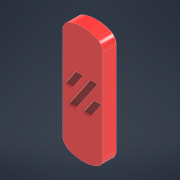
# Autodesk Inventor part: Cover_Square
Saved by Autodesk Inventor 2022.1 (Build 261234000, 234)
## iProperties
Created: 2021-09-01
Part Number: Cover_Square
Material: Generisch
Document SubType Name: Modeling
Designer: Rama
Density: 1 g/cm^3
Appearance: Hellrot
Author: Rama
Autodesk Inventor part; units mm, degrees
ref_plane "YZ Plane" through (0, 0, 0) normal (1, 0, 0) x (0, 1, 0)
ref_plane "XZ Plane" through (0, 0, 0) normal (0, 1, 0) x (-1, 0, 0)
sketch "Skizze1" plane through (0, 0, 0) normal (0, 0, 1) x (1, 0, 0)
  line L0 (7.75, -17.6806) -> (7.75, 17.6806) projected
  line L1 (-7.75, 17.6806) -> (-7.75, -17.6806) projected
  circle A0 centre (0, 0) radius 3.025 projected
  arc A1 (-5.3363, -21.3526) -> (5.3363, -21.3526) centre (0, -9) ccw projected
  arc A2 (5.3363, -21.3526) -> (7.75, -17.6806) centre (3.75, -17.6806) ccw projected
  arc A3 (7.75, 17.6806) -> (5.3363, 21.3526) centre (3.75, 17.6806) ccw projected
  arc A4 (5.3363, 21.3526) -> (-5.3363, 21.3526) centre (0, 9) ccw projected
  arc A5 (-5.3363, 21.3526) -> (-7.75, 17.6806) centre (-3.75, 17.6806) ccw projected
  arc A6 (-7.75, -17.6806) -> (-5.3363, -21.3526) centre (-3.75, -17.6806) ccw projected
  circle A7 centre (-0.25, 17) radius 1.7 projected
  circle A8 centre (-0.25, -7) radius 1.7 projected
  line L2 (5.34, 14.1) -> (3.3, 14.1) projected
  line L3 (3.3, 14.1) -> (3.3, 17.74) projected
  line L4 (3.3, 17.74) -> (5.34, 17.74) projected
  line L5 (5.34, 17.74) -> (5.34, 14.1) projected
  line L6 (-3.8, 14.1) -> (-5.84, 14.1) projected
  line L7 (-5.84, 14.1) -> (-5.84, 17.74) projected
  line L8 (-5.84, 17.74) -> (-3.8, 17.74) projected
  line L9 (-3.8, 17.74) -> (-3.8, 14.1) projected
  circle A9 centre (-0.25, -15.278) radius 2.9 projected
  point P0 (0, 0)
  point P1 (-17.1225, -5.975)
  point P2 (-17.1225, -12.025)
  point P3 (-17.1225, 6.3)
  point P4 (-17.1225, -14.3)
  point P5 (-17.1225, -17.7)
  constraints: 1 other
extrude "Extrusion1" add sketch "Skizze1" along normal blind 4 contours A2 A1 A6 L1 A5 A4 A3 L0 | A0 | A7 | A8 | L2 L3 L4 L5 | L6 L7 L8 L9 | A9
sketch "Skizze2" plane through (0, 0, 0) normal (0, 0, -1) x (-1, 0, 0)
  circle A0 centre (0, 0) radius 3.025 projected
  arc A1 (-5.3363, -21.3526) -> (5.3363, -21.3526) centre (0, -9) ccw projected
  arc A2 (-7.75, -17.6806) -> (-5.3363, -21.3526) centre (-3.75, -17.6806) ccw projected
  line L0 (-7.75, -17.6806) -> (-7.75, 17.6806) projected
  arc A3 (-5.3363, 21.3526) -> (-7.75, 17.6806) centre (-3.75, 17.6806) ccw projected
  arc A4 (5.3363, 21.3526) -> (-5.3363, 21.3526) centre (0, 9) ccw projected
  arc A5 (7.75, 17.6806) -> (5.3363, 21.3526) centre (3.75, 17.6806) ccw projected
  line L1 (7.75, 17.6806) -> (7.75, -17.6806) projected
  arc A6 (5.3363, -21.3526) -> (7.75, -17.6806) centre (3.75, -17.6806) ccw projected
  circle A7 centre (0.25, 17) radius 1.7 projected
  circle A8 centre (0.25, -7) radius 1.7 projected
  line L2 (-5.34, 14.1) -> (-3.3, 14.1) projected
  line L3 (-3.3, 14.1) -> (-3.3, 17.74) projected
  line L4 (-3.3, 17.74) -> (-5.34, 17.74) projected
  line L5 (-5.34, 17.74) -> (-5.34, 14.1) projected
  line L6 (3.8, 14.1) -> (5.84, 14.1) projected
  line L7 (5.84, 14.1) -> (5.84, 17.74) projected
  line L8 (5.84, 17.74) -> (3.8, 17.74) projected
  line L9 (3.8, 17.74) -> (3.8, 14.1) projected
  circle A9 centre (0.25, -15.278) radius 2.9 projected
  point P0 (0, 0)
extrude "Extrusion2" cut sketch "Skizze2" against normal blind 3.1 contours A0
sketch "Skizze3" plane through (0, 0, 0) normal (0, 0, -1) x (-1, 0, 0)
  circle A0 centre (0, 0) radius 3.025 projected
  arc A1 (-5.3363, -21.3526) -> (5.3363, -21.3526) centre (0, -9) ccw projected
  arc A2 (-7.75, -17.6806) -> (-5.3363, -21.3526) centre (-3.75, -17.6806) ccw projected
  line L0 (-7.75, -17.6806) -> (-7.75, 17.6806) projected
  arc A3 (-5.3363, 21.3526) -> (-7.75, 17.6806) centre (-3.75, 17.6806) ccw projected
  arc A4 (5.3363, 21.3526) -> (-5.3363, 21.3526) centre (0, 9) ccw projected
  arc A5 (7.75, 17.6806) -> (5.3363, 21.3526) centre (3.75, 17.6806) ccw projected
  line L1 (7.75, 17.6806) -> (7.75, -17.6806) projected
  arc A6 (5.3363, -21.3526) -> (7.75, -17.6806) centre (3.75, -17.6806) ccw projected
  circle A7 centre (0.25, 17) radius 1.7 projected
  circle A8 centre (0.25, -7) radius 1.7 projected
  line L2 (-5.34, 14.1) -> (-3.3, 14.1) projected
  line L3 (-3.3, 14.1) -> (-3.3, 17.74) projected
  line L4 (-3.3, 17.74) -> (-5.34, 17.74) projected
  line L5 (-5.34, 17.74) -> (-5.34, 14.1) projected
  line L6 (3.8, 14.1) -> (5.84, 14.1) projected
  line L7 (5.84, 14.1) -> (5.84, 17.74) projected
  line L8 (5.84, 17.74) -> (3.8, 17.74) projected
  line L9 (3.8, 17.74) -> (3.8, 14.1) projected
  circle A9 centre (0.25, -15.278) radius 2.9 projected
  point P0 (0, 0)
hole "Bohrung1" at (-0.25, 17, 0) at (-0.25, -7, 0) direction (0, 0, 1) diameter 5.6 depth 3.2 counterbore diameter 7.1 counterbore depth 1.2
sketch "Skizze4" plane through (0, 0, 4) normal (0, 0, 1) x (1, 0, 0)
  circle A0 centre (-0.25, 17) radius 3.55 projected
  circle A1 centre (-0.25, -7) radius 3.55 projected
  circle A2 centre (0, 0) radius 3.025 projected
  arc A3 (5.3363, -21.3526) -> (7.75, -17.6806) centre (3.75, -17.6806) ccw projected
  arc A4 (-5.3363, -21.3526) -> (5.3363, -21.3526) centre (0, -9) ccw projected
  arc A5 (-7.75, -17.6806) -> (-5.3363, -21.3526) centre (-3.75, -17.6806) ccw projected
  line L0 (-7.75, 17.6806) -> (-7.75, -17.6806) projected
  arc A6 (-5.3363, 21.3526) -> (-7.75, 17.6806) centre (-3.75, 17.6806) ccw projected
  arc A7 (5.3363, 21.3526) -> (-5.3363, 21.3526) centre (0, 9) ccw projected
  arc A8 (7.75, 17.6806) -> (5.3363, 21.3526) centre (3.75, 17.6806) ccw projected
  line L1 (7.75, -17.6806) -> (7.75, 17.6806) projected
  circle A9 centre (12.6079, -10) radius 2.8
  circle A10 centre (12.6079, -10) radius 2.8
  line L2 (4.1087, 0) -> (7.1087, 0)
  line L3 (7.1087, 0) -> (2.8877, -6.1994)
  line L4 (2.8877, -6.1994) -> (-0.1123, -6.1994)
  line L5 (-0.1123, -6.1994) -> (4.1087, 0)
  line L6 (2.721, 6.1994) -> (5.721, 6.1994)
  line L7 (5.721, 6.1994) -> (-2.721, -6.1994)
  line L8 (-2.721, -6.1994) -> (-5.721, -6.1994)
  line L9 (-5.721, -6.1994) -> (2.721, 6.1994)
  line L10 (-2.8877, 6.1994) -> (0.1123, 6.1994)
  line L11 (0.1123, 6.1994) -> (-4.1087, 0)
  line L12 (-4.1087, 0) -> (-7.1087, 0)
  line L13 (-7.1087, 0) -> (-2.8877, 6.1994)
  line L14 (7.1087, 6.1994) -> (7.1087, -6.1994)
  line L15 (7.1087, -6.1994) -> (-7.1087, -6.1994)
  line L16 (-7.1087, -6.1994) -> (-7.1087, 6.1994)
  line L17 (-7.1087, 6.1994) -> (7.1087, 6.1994)
  point P0 (0, 0)
  point P1 (16.5579, -10)
  point P2 (16.5579, -10)
  point P3 (16.5579, -10)
  point P4 (50.5428, -9.282)
  point P5 (-4.221, -6.1994)
  point P6 (4.221, 6.1994)
  point P7 (-1.3877, 6.1994)
  point P8 (1.3877, -6.1994)
  dimension "d89" = 5.6
  dimension "d104" = 5.6
  dimension "d107" = 14.2174
  dimension "d108" = 12.3988
  dimension "d109" = 2.1563
  dimension "d110" = 2.1563
  dimension "d111" = 2.4798
  dimension "d112" = 2.4798
  dimension "d113" = 2.4798
  dimension "d114" = 6.1994
  dimension "d115" = 6.1994
  dimension "d116" = 6.1994
  dimension "d117" = 15.5
  dimension "d118" = 0.6413
  constraints: 32 end point, 6 midpoint, 4 point on line, 2 centre point, 2 coincident, 2 parallel, 1 perpendicular
  measures "d89" diameter of A9
  measures "d104" diameter of A10
  measures "d107" distance between parallel lines of L14 L16
  measures "d108" distance between parallel lines of L15 L17
  measures "d109" distance between parallel lines of L7 L5
  measures "d110" distance between parallel lines of L11 L9
  measures "d111" distance between parallel lines of L9 L7
  measures "d112" distance between parallel lines of L5 L3
  measures "d113" distance between parallel lines of L13 L11
  measures "d114" distance between parallel lines of L15 L2
  measures "d115" distance between parallel lines of L17 L12
  measures "d116" distance from line of point (0, 0) L15
  measures "d117" distance between parallel lines of L1 L0
  measures "d118" distance between parallel lines of L0 L16
move faces "Verschieben1" translate (0, 0, 0.5) faces at (-2.5833, -5.8935, 4)
fillet "Rundung2" radius 3.5 8 edges at (-7.0925, -19.8777, 4.5) (0, -22.4559, 4.5) (7.0925, -19.8777, 4.5) (7.75, 0, 4.5) (7.0925, 19.8777, 4.5) (0, 22.4559, 4.5) (-7.0925, 19.8777, 4.5) (-7.75, 0, 4.5)
extrude "Extrusion4" cut sketch "Skizze4" along normal mid plane 0.8 contours L8 L9 A2 L7 A1 | A1 L7 L8 | L3 L4 L5 A1 | A1 L5 L2 L3 | A2 L9 L7 | A2 L9 L6 L7 | L13 L10 L11 L12
extrude "Extrusion5" cut sketch "Skizze4" along normal through all contours L8 L9 A2 L7 A1 | A1 L7 L8 | L3 L4 L5 A1 | A1 L5 L2 L3 | A2 L9 L7 | A2 L9 L6 L7 | L13 L10 L11 L12
sketch "Skizze5" plane through (0, 0, 0) normal (0, 0, -1) x (-1, 0, 0)
  circle A0 centre (0.25, -15.278) radius 2.9 projected
  point P0 (0, 0)
extrude "Extrusion6" cut sketch "Skizze5" against normal blind 1.4
move faces "Verschieben2" translate (0, 0, -1) faces at (6.175, 0, 0)
move faces "Verschieben4" translate (0, 0, -1.5) faces at (0.2566, 20.2385, 1.2) (0.3195, 20.504, 0.4667) (0.1992, 19.7637, 2.5333) (-1.1227, 17.331, 3.2) (0.2566, -3.7615, 1.2) (0.3195, -3.496, 0.4667) (0.1992, -4.2363, 2.5333) (-0.6585, -8.034, 3.2)
move faces "Verschieben5" translate (0, 0, -1) faces at (0.0815, -15.3652, 1.4)
chamfer "Fase11" distance 0.4 angle 45 8 edges at (7.75, 0, -1) (7.0925, 19.8777, -1) (0, 22.4559, -1) (-7.0925, 19.8777, -1) (-7.75, 0, -1) (-7.0925, -19.8777, -1) (0, -22.4559, -1) (7.0925, -19.8777, -1)
ref_plane "Arbeitsebene1" through (-0.25, 17, 1.7) normal (0, 0, -1) x (-1, 0, 0)
sketch "Skizze6" plane through (-0.25, 17, 1.7) normal (0, 0, -1) x (-1, 0, 0)
  circle A0 centre (0, 0) radius 2 projected
  circle A1 centre (0, -24) radius 2 projected
  circle A2 centre (0, 0) radius 2.4
  circle A3 centre (0, -24) radius 2.4
  point P0 (-0.25, -17)
  dimension "d176" = 4.8
  dimension "d177" = 4.8
  constraints: 2 centre point, 2 coincident
  measures "d176" diameter of A2
  measures "d177" diameter of A3
extrude "Extrusion7" cut sketch "Skizze6" along normal through all contours A0 | A1 | A2 | A3
move faces "Verschieben6" translate (0, 0, -0.75) faces at (0.4956, 0.1944, 3.1)
sketch "Skizze7" plane through (0, -9, -1) normal (0, 0, -1) x (-1, 0, 0)
  line L0 (7.35, 26.6806) -> (7.35, -8.6806) projected
  line L1 (4.25, 13.1986) -> (4.25, 26.6806) projected
  circle A0 centre (0, 9) radius 3.025 projected
  circle A1 centre (0.25, 2) radius 3.55 projected
  circle A2 centre (0.25, 26) radius 3.55 projected
  circle A3 centre (0.25, -6.278) radius 2.9 projected
  line L2 (-7.35, -8.6806) -> (-7.35, 26.6806) projected
  arc A4 (-7.35, -8.6806) -> (-5.1777, -11.9854) centre (-3.75, -8.6806) ccw projected
  arc A5 (-5.1777, -11.9854) -> (5.1777, -11.9854) centre (0, 0) ccw projected
  arc A6 (5.1777, -11.9854) -> (7.35, -8.6806) centre (3.75, -8.6806) ccw projected
  line L3 (7.35, 26.6806) -> (7.35, -8.6806) projected
  arc A7 (7.35, 26.6806) -> (5.1777, 29.9854) centre (3.75, 26.6806) ccw projected
  arc A8 (5.1777, 29.9854) -> (-5.1777, 29.9854) centre (0, 18) ccw projected
  arc A9 (-5.1777, 29.9854) -> (-7.35, 26.6806) centre (-3.75, 26.6806) ccw projected
  point P0 (0, 9)
hole "Bohrung2" at (-0.25, 17, -1) at (-0.25, -7, -1) direction (0, 0, 1) diameter 6.5 depth 4 counterbore diameter 7.5 counterbore depth 1.4
chamfer "Fase12" distance 0.5 angle 45 1 edges at (-0.25, -10.25, 0.4)
sketch "Skizze8" plane through (-0.25, -7, 3) normal (0, 0, -1) x (-1, 0, 0)
  circle A0 centre (0, 0) radius 3.25 projected
  circle A1 centre (0, 24) radius 3.25 projected
  circle A2 centre (0, 24) radius 3.25 projected
  line L0 (0, 27.25) -> (0, 20.75)
  circle A3 centre (0, 0) radius 3.25 projected
  line L1 (0, 3.25) -> (0, -3.25)
  point P0 (-0.25, 7)
  point P1 (0, 3.25)
  point P2 (0, -3.25)
  constraints: 4 end point, 4 point on circle, 2 point on line, 1 vertical
extrude "Extrusion8" add sketch "Skizze8" along normal blind 0.2 contours A0 L1 | A1 L0 picked at (1.7635, -0.8846) picked at (1.694, 22.9167)
delete faces "Fläche löschen3" heal yes whole lump no faces at (7.7109, 5.8935, 1.5216) (6.4358, 20.5252, 1.7788) (7.4265, -19.018, 1.7788) (1.8221, 22.3221, 1.2616) (-3.6106, -21.9523, 1.2616) (-6.4358, 20.5252, 1.7788) (-7.4265, -19.018, 1.7788) (-7.5945, 5.8935, 2.0316)
